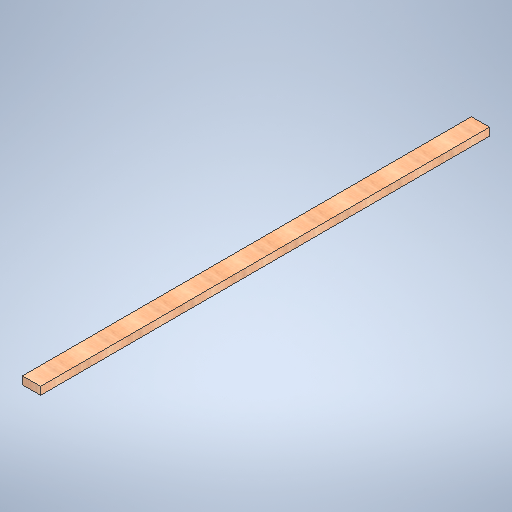
# Autodesk Inventor part: Plate_With_Length_90.75_Inches
Saved by Autodesk Inventor 2025 (Build 290162010, 162A)
## iProperties
Created: 2024-09-20
Part Number: Plate_With_Length_90.75_Inches
Material: Wood (Birch)
Document SubType Name: Modeling
Designer: Tom
Density: 0.55 g/cm^3
Appearance: Birch - Natural Polished
Author: Tom
Autodesk Inventor part; units mm, degrees
ref_plane "YZ Plane" through (0, 0, 0) normal (1, 0, 0) x (0, 1, 0)
ref_plane "XZ Plane" through (0, 0, 0) normal (0, 1, 0) x (-1, 0, 0)
ref_plane "XY Plane" through (0, 0, 0) normal (0, 0, 1) x (1, 0, 0)
sketch "Sketch1" plane through (0, 0, 0) normal (0, 1, 0) x (-1, 0, 0)
  line L0 (0, 0) -> (88.9, 0)
  line L1 (88.9, 0) -> (88.9, -2198.6875)
  line L2 (88.9, -2198.6875) -> (0, -2198.6875)
  line L3 (0, -2198.6875) -> (0, 0)
  dimension "d1" = 88.9
  dimension "d4" = 2198.6875
  constraints: 8 end point, 2 parallel, 1 horizontal, 1 perpendicular
  measures "d1" distance of L0.start L0.end
  measures "d4" distance of L2.end L0.start
extrude "Extrusion1" add sketch "Sketch1" along normal blind 38.1
sketch "Sketch2" plane through (-88.9, 0, -2198.6875) normal (-1, 0, 0) x (0, 0, 1)
  line L0 (0, 423.1077) -> (739.775, 423.1077) construction
  line L1 (739.775, 423.1077) -> (739.775, -68.2625) construction
  line L2 (739.775, -68.2625) -> (0, -68.2625) construction
  line L3 (0, -68.2625) -> (0, 423.1077) construction
  line L4 (0, 0) -> (0, 38.1) projected
  line L5 (0, 0) -> (2198.6875, 0) projected
  dimension "d6" = 739.775
  dimension "d14" = 68.2625
  constraints: 1 collinear, 2 other
  measures "d6" distance of L0.start L0.end
  measures "d14" distance between parallel lines of L5 L2
body "Solid1"
